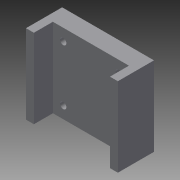
# Autodesk Inventor part: sbr20uu_standoff
Saved by Autodesk Inventor 2014 (Build 180170000, 170)
## iProperties
Created: 2014-10-03
Part Number: sbr20uu_standoff
Material: Generic
Document SubType Name: Modeling
Designer: Matthew
Density: 1 g/cm^3
Appearance: Default
Author: Matthew
Autodesk Inventor part; units mm, degrees
ref_plane "YZ Plane" through (0, 0, 0) normal (1, 0, 0) x (0, 1, 0)
ref_plane "XZ Plane" through (0, 0, 0) normal (0, 1, 0) x (-1, 0, 0)
ref_plane "XY Plane" through (0, 0, 0) normal (0, 0, 1) x (1, 0, 0)
sketch "Sketch1" plane through (0, 0, 0) normal (0, 1, 0) x (-1, 0, 0)
  line L0 (29, -25) -> (-29, -25)
  line L1 (-29, -25) -> (-29, 25)
  line L2 (-29, 25) -> (29, 25)
  line L3 (29, 25) -> (29, -25)
  line L4 (29, -25) -> (-29, 25) construction
  line L5 (-29, -25) -> (29, 25) construction
  point P0 (0, 0)
  dimension "d0" = 58
  dimension "d1" = 50
  constraints: 12 end point, 2 midpoint, 2 parallel, 1 horizontal, 1 perpendicular
  measures "d0" distance of L1.end L2.end
  measures "d1" distance of L0.end L1.end
extrude "Extrusion1" add sketch "Sketch1" along normal blind 10.8204
sketch "Sketch2" plane through (0, 0, 0) normal (0, -1, 0) x (1, 0, 0)
  line L0 (-29, -25) -> (29, -25) projected
  line L1 (29, -25) -> (29, 25) projected
  line L2 (29, 25) -> (-29, 25) projected
  line L3 (-29, 25) -> (-29, -25) projected
  line L4 (-24, 25) -> (-24, -25)
  line L5 (24, 25) -> (24, -25)
  point P0 (0, 0)
  dimension "d4" = 5
  dimension "d5" = 5
  constraints: 4 end point, 4 point on line, 2 perpendicular
  measures "d4" distance between parallel lines of L1 L5
  measures "d5" distance between parallel lines of L3 L4
extrude "Extrusion2" add sketch "Sketch2" along normal blind 12 contours L3 L2 L4 L0 | L5 L2 L1 L0
sketch "Sketch3" plane through (0, 10.8204, 0) normal (0, 1, 0) x (1, 0, 0)
  line L0 (29, 25) -> (-29, 25) projected
  line L1 (-29, 25) -> (-29, -25) projected
  point P0 (0, 0)
  point P1 (-17.5, 17.5)
  point P2 (17.5, 17.5)
  point P3 (-17.5, -17.5)
  point P4 (17.5, -17.5)
  dimension "d10" = 35
  dimension "d13" = 35
  dimension "d16" = 11.5
  dimension "d17" = 58
  dimension "d18" = 50
  dimension "d19" = 7.5
  constraints: 1 horizontal, 1 vertical, 3 other
  measures "d10" distance of point (-17.5, 17.5) point (17.5, 17.5)
  measures "d13" distance of point (-17.5, 17.5) point (-17.5, -17.5)
  measures "d16" distance from line of L1 point (-17.5, 17.5)
  measures "d17" distance of L0.start L0.end
  measures "d18" distance of L0.end L1.end
  measures "d19" distance from line of L0 point (-17.5, 17.5)
hole "Hole1" at (-17.5, 10.8204, -17.5) at (17.5, 10.8204, -17.5) at (-17.5, 10.8204, 17.5) at (17.5, 10.8204, 17.5) direction (0, -1, 0) diameter 4 end through all
equation "\"d5\" = d4"
equation "\"d16\" = -0.5 * d10 + 0.5 * d17"
equation "\"d19\" = -0.5 * d13 + 0.5 * d18"
body "Solid1"
